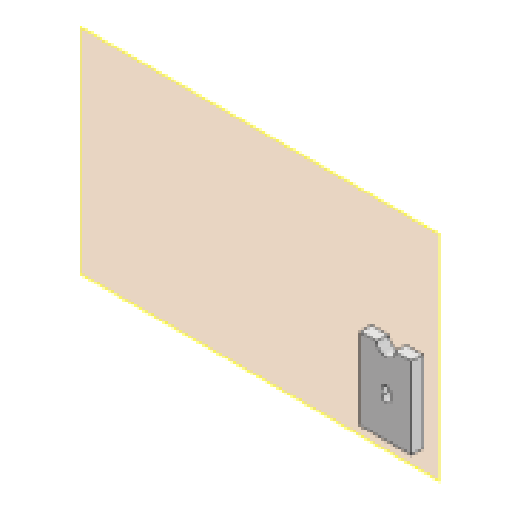
# Autodesk Inventor part: Cuvette Aligner 10mm
Saved by Autodesk Inventor 2025.1 (Build 291241020, 241B)
## iProperties
Created: 2024-09-24
Part Number: Cuvette Aligner 10mm
Material: Generic
Document SubType Name: Modeling
Designer: wayneslade
Density: 1 g/cm^3
Appearance: Default
Author: wayneslade
Autodesk Inventor part; units mm, degrees
ref_plane "YZ Plane" through (0, 0, 0) normal (1, 0, 0) x (0, 1, 0)
ref_plane "XZ Plane" through (0, 0, 0) normal (0, 1, 0) x (-1, 0, 0)
ref_plane "XY Plane" through (0, 0, 0) normal (0, 0, 1) x (1, 0, 0)
ref_plane "Work Plane1" through (0, 0, 0) normal (0, 0, 1) x (1, 0, 0)
sketch "Sketch1" plane through (0, 0, 0) normal (0, 0, 1) x (1, 0, 0)
  circle A0 centre (11.5562, -18) radius 2 construction
  line L0 (-53.1938, -16) -> (-53.1938, -30) construction
  arc A1 (-56.1938, -30) -> (-53.1938, -30) centre (-54.6938, -30) ccw construction
  line L1 (-56.1938, -30) -> (-56.1938, -16) construction
  arc A2 (-53.1938, -16) -> (-56.1938, -16) centre (-54.6938, -16) ccw construction
  line L2 (7.0562, -16) -> (7.0562, -30) construction
  arc A3 (4.0562, -30) -> (7.0562, -30) centre (5.5562, -30) ccw construction
  line L3 (4.0562, -30) -> (4.0562, -16) construction
  arc A4 (7.0562, -16) -> (4.0562, -16) centre (5.5562, -16) ccw construction
  line L4 (-13.1938, -16) -> (-13.1938, -30) construction
  arc A5 (-16.1938, -30) -> (-13.1938, -30) centre (-14.6938, -30) ccw construction
  line L5 (-16.1938, -30) -> (-16.1938, -16) construction
  arc A6 (-13.1938, -16) -> (-16.1938, -16) centre (-14.6938, -16) ccw construction
  arc A7 (19.0562, -16) -> (16.0562, -16) centre (17.5562, -16) ccw construction
  line L6 (19.0562, -16) -> (19.0562, -30) construction
  arc A8 (16.0562, -30) -> (19.0562, -30) centre (17.5562, -30) ccw construction
  line L7 (16.0562, -30) -> (16.0562, -16) construction
  line L8 (22.8064, -40) -> (22.8064, 45) construction
  line L9 (22.8064, 45) -> (-120, 45) construction
  line L10 (-120, 27.5563) -> (-120, 45) construction
  line L11 (-120, 27.5563) -> (-95.2035, 27.5563) construction
  arc A9 (-85.0841, 27.5563) -> (-95.2035, 27.5563) centre (-90.1438, 25.4) ccw construction
  line L12 (-85.0841, 27.5563) -> (17.8062, 27.5563) construction
  line L13 (17.8062, 27.5563) -> (17.8062, -11) construction
  line L14 (17.8062, -11) -> (-120, -11) construction
  line L15 (-120, -40) -> (-120, -11) construction
  line L16 (22.8064, -40) -> (-120, -40) construction
  circle A10 centre (-111.1938, -18) radius 2 construction
  circle A11 centre (-98.1938, -18) radius 2 construction
  circle A12 centre (-61.1938, -18) radius 2 construction
  circle A13 centre (-48.1938, -18) radius 2 construction
  circle A14 centre (-21.1938, -18) radius 2 construction
  circle A15 centre (-8.1938, -18) radius 2 construction
  circle A16 centre (-21.1938, 33.6563) radius 2 construction
  circle A17 centre (-8.1938, 33.6563) radius 2 construction
  circle A18 centre (-61.1938, 33.6563) radius 2 construction
  circle A19 centre (-48.1938, 33.6563) radius 2 construction
  circle A20 centre (-111.1938, 33.6563) radius 2 construction
  circle A21 centre (-98.1938, 33.6563) radius 2 construction
  circle A22 centre (-90.1438, -25.4) radius 5.5 construction
  line L17 (5.3062, -11) -> (5.3062, 11) construction
  line L18 (17.8062, -11) -> (17.8062, 11) construction
  circle A23 centre (11.5562, 0) radius 3.75 construction
  line L19 (5.3062, -11) -> (17.8062, -11) construction
  arc A24 (-18.6938, -19.75) -> (-18.6938, -16.25) centre (-18.6938, -18) ccw construction
  line L20 (-18.6938, -16.25) -> (-23.6938, -16.25) construction
  arc A25 (-23.6938, -16.25) -> (-23.6938, -19.75) centre (-23.6938, -18) ccw construction
  line L21 (-23.6938, -19.75) -> (-18.6938, -19.75) construction
  arc A26 (-5.6938, -19.75) -> (-5.6938, -16.25) centre (-5.6938, -18) ccw construction
  line L22 (-5.6938, -16.25) -> (-10.6938, -16.25) construction
  arc A27 (-10.6938, -16.25) -> (-10.6938, -19.75) centre (-10.6938, -18) ccw construction
  line L23 (-10.6938, -19.75) -> (-5.6938, -19.75) construction
  line L24 (0.3062, -11) -> (0.3062, -25.3437) construction
  line L25 (0.3062, -25.3437) -> (-29.6938, -25.3437) construction
  line L26 (-29.6938, -11) -> (-29.6938, -25.3437) construction
  line L27 (0.3062, -11) -> (-29.6938, -11) construction
  line L28 (22.8064, -35.5) -> (0.3062, -35.5)
  line L29 (0.3062, -35.5) -> (0.3062, 0)
  line L30 (0.3062, 0) -> (7.7062, 0)
  line L31 (22.8064, 0) -> (22.8064, -35.5)
  arc A28 (7.7062, 0) -> (15.4062, 0) centre (11.5562, 0) ccw
  line L32 (11.5562, 15.4) -> (11.5562, -15.4) construction
  line L33 (-148.5613, 0) -> (51.3677, 0) construction
  line L34 (15.4062, 0) -> (22.8064, 0)
  point P0 (0, 0)
  point P1 (17.5562, -31.5)
  dimension "d0" = 0.1
  dimension "d1" = 0
  dimension "d2" = 0
  dimension "d3" = 4
  constraints: 14 end point, 3 parallel, 3 point on circle, 2 collinear, 2 horizontal, 1 centre point, 1 coincident, 1 perpendicular, 1 point on line, 1 vertical, 2 other
  measures "d0" radial gap between concentric circles of A23 A28
  measures "d1" distance between parallel lines of L8 L31
  measures "d2" distance between parallel lines of L24 L29
  measures "d3" distance from line of L28 point (17.556, -31.5)
extrude "Main Body" add sketch "Sketch1" along normal blind 5
sketch "Sketch2" plane through (0, 0, 0) normal (0, 0, -1) x (-1, 0, 0)
  line L0 (-16.0562, -30) -> (-16.0562, -16) construction
  arc A0 (-19.0562, -30) -> (-16.0562, -30) centre (-17.5562, -30) ccw construction
  line L1 (-19.0562, -16) -> (-19.0562, -30) construction
  arc A1 (-16.0562, -16) -> (-19.0562, -16) centre (-17.5562, -16) ccw construction
  arc A2 (-7.0562, -30) -> (-4.0562, -30) centre (-5.5562, -30) ccw construction
  line L2 (-7.0562, -16) -> (-7.0562, -30) construction
  arc A3 (-4.0562, -16) -> (-7.0562, -16) centre (-5.5562, -16) ccw construction
  line L3 (-4.0562, -30) -> (-4.0562, -16) construction
  line L4 (-17.5562, -30) -> (-17.5562, -16) construction
  line L5 (-5.5562, -16) -> (-5.5562, -30) construction
  line L6 (-17.5562, -29) -> (-17.5562, -17) construction
  line L7 (-16.1062, -29) -> (-16.1062, -17)
  line L8 (-19.0062, -17) -> (-19.0062, -29)
  arc A4 (-19.0062, -29) -> (-16.1062, -29) centre (-17.5562, -29) ccw
  arc A5 (-16.1062, -17) -> (-19.0062, -17) centre (-17.5562, -17) ccw
  line L9 (-5.5562, -29) -> (-5.5562, -17) construction
  line L10 (-4.1062, -29) -> (-4.1062, -17)
  line L11 (-7.0062, -17) -> (-7.0062, -29)
  arc A6 (-7.0062, -29) -> (-4.1062, -29) centre (-5.5562, -29) ccw
  arc A7 (-4.1062, -17) -> (-7.0062, -17) centre (-5.5562, -17) ccw
  line L12 (-17.5562, -29) -> (-5.5562, -29) construction
  line L13 (-17.5562, -17) -> (-5.5562, -17) construction
  point P0 (0, 0)
  point P1 (-17.5562, -23)
  point P2 (-5.5562, -23)
  dimension "d6" = 1
  dimension "d7" = 0.05
  dimension "d8" = 0.05
  constraints: 24 end point, 8 point on circle, 8 tangent, 4 centre point, 4 midpoint, 2 parallel, 2 point on line, 1 horizontal, 1 vertical
  measures "d6" distance of L6.start L4.start
  measures "d7" distance between parallel lines of L1 L8
  measures "d8" distance between parallel lines of L2 L11
extrude "Alignment Tabs" add sketch "Sketch2" along normal blind 1.8
sketch "Sketch3" plane through (0, 0, 5) normal (0, 0, 1) x (1, 0, 0)
  circle A0 centre (11.5562, -18) radius 2 construction
  line L0 (11.5562, -19.5) -> (11.5562, -16.5) construction
  line L1 (13.3062, -19.5) -> (13.3062, -16.5)
  line L2 (9.8062, -16.5) -> (9.8062, -19.5)
  arc A1 (9.8062, -19.5) -> (13.3062, -19.5) centre (11.5562, -19.5) ccw
  arc A2 (13.3062, -16.5) -> (9.8062, -16.5) centre (11.5562, -16.5) ccw
  point P0 (0, 0)
  dimension "d11" = 3.5
  dimension "d12" = 3
  constraints: 8 end point, 4 point on circle, 4 tangent, 2 centre point, 1 midpoint, 1 parallel, 1 vertical
  measures "d11" distance between parallel lines of L2 L1
  measures "d12" distance of L0.end L0.start
extrude "Slot for Screw M3" cut sketch "Sketch3" against normal through all
equation "\"d8\" = d7"
body "Solid1"
